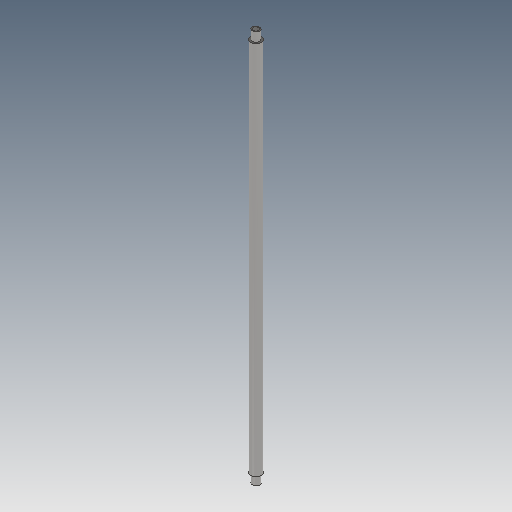
# Autodesk Inventor part: Guias de mesa
Saved by Autodesk Inventor 2020.3 (Build 243373000, 373)
## iProperties
Created: 2020-05-08
Part Number: Guias de mesa
Material: Steel, High Strength, Low Alloy
Document SubType Name: Modeling
Designer: Pipi
Density: 7.85 g/cm^3
Appearance: Steel - Polished
Mass: 374.835 g
Surface Area: 170.117 cm^2
Volume: 47.7496 cm^3
Author: Pipi
Autodesk Inventor part; units mm, degrees
ref_plane "YZ Plane" through (0, 0, 0) normal (1, 0, 0) x (0, 1, 0)
ref_plane "XZ Plane" through (0, 0, 0) normal (0, 1, 0) x (-1, 0, 0)
ref_plane "XY Plane" through (0, 0, 0) normal (0, 0, 1) x (1, 0, 0)
sketch "Boceto1" plane through (0, 0, 0) normal (0, 1, 0) x (-1, 0, 0)
  circle A0 centre (4.6883, 13.1099) radius 6
  point P0 (0, 0)
  dimension "d0" = 12
  constraints: 1 centre point
  measures "d0" diameter of A0
extrude "Extrusión1" add sketch "Boceto1" along normal blind 434
sketch "Boceto2" plane through (-4.6883, 434, 13.1099) normal (0, 1, 0) x (1, 0, 0)
  circle A0 centre (0, 0) radius 3
  point P0 (4.6883, 13.1099)
  dimension "d3" = 6
  constraints: 1 centre point
  measures "d3" diameter of A0
hole "Agujero1" at (-4.6883, 434, 13.1099) direction (0, -1, 0) diameter 6 depth 15 tip angle 118
sketch "Boceto3" plane through (-4.6883, 0, 13.1099) normal (0, -1, 0) x (1, 0, 0)
  circle A0 centre (0, 0) radius 3
  point P0 (4.6883, -13.1099)
  dimension "d11" = 6
  constraints: 1 centre point
  measures "d11" diameter of A0
hole "Agujero2" at (-4.6883, 0, 13.1099) direction (0, 1, 0) diameter 6 depth 15 tip angle 118
thread "Thread1" size "M6x1" class "6H" standard "ANSI Metric M Profile" length 40
thread "Thread2" size "M6x1" class "6H" standard "ANSI Metric M Profile" length 40
sketch "Boceto4" plane through (-4.6883, 434, 13.1099) normal (0, 1, 0) x (1, 0, 0)
  circle A0 centre (0, 0) radius 4
  circle A1 centre (0, 0) radius 6
  point P0 (4.6883, 13.1099)
  dimension "d23" = 8
  constraints: 2 centre point, 1 coincident
  measures "d23" diameter of A0
sketch "Boceto5" plane through (-4.6883, 0, 13.1099) normal (0, -1, 0) x (1, 0, 0)
  circle A0 centre (0, 0) radius 4
  circle A1 centre (0, 0) radius 6
  point P0 (4.6883, -13.1099)
  dimension "d24" = 8
  constraints: 2 centre point, 1 coincident
  measures "d24" diameter of A0
extrude "Extrusión2" cut sketch "Boceto5" against normal blind 10
extrude "Extrusión3" cut sketch "Boceto4" against normal blind 10
